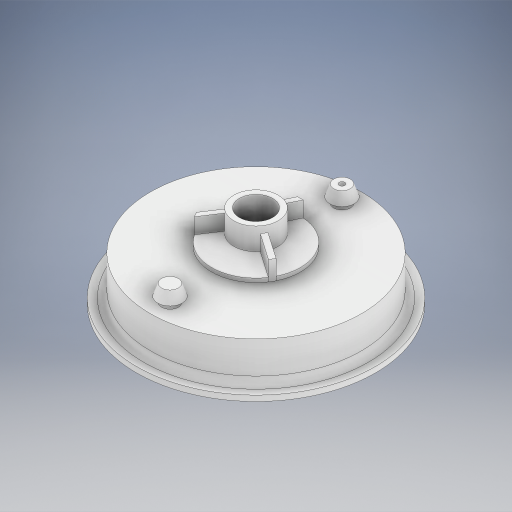
# Autodesk Inventor part: Pressure Plate
Saved by Autodesk Inventor 2024.1 (Build 281209000, 209)
## iProperties
Created: 2023-11-09
Part Number: Pressure Plate
Material: Acetal Resin, White
Document SubType Name: Modeling
Designer: Glen Collingwood
Density: 1.425 g/cm^3
Appearance: Smooth - White
Author: Glen Collingwood
Autodesk Inventor part; units mm, degrees
ref_plane "YZ Plane" through (0, 0, 0) normal (1, 0, 0) x (0, 1, 0)
ref_plane "XZ Plane" through (0, 0, 0) normal (0, 1, 0) x (-1, 0, 0)
ref_plane "XY Plane" through (0, 0, 0) normal (0, 0, 1) x (1, 0, 0)
sketch "Sketch1" plane through (0, 0, 0) normal (1, 0, 0) x (0, 1, 0)
  line L0 (0, 0) -> (0.5, 0)
  line L1 (0.5, 0) -> (0.5, -9.5)
  line L2 (0.5, -9.5) -> (0, -9.5)
  line L3 (0, -9.5) -> (0, 0)
  line L4 (0, 0) -> (-3.6315, 0)
  line L5 (0, -9.5) -> (-2.4, -9.5)
  line L6 (-3.5, -9.5) -> (-3.5, -9)
  line L7 (-2.4, -9) -> (0, -9)
  line L8 (0, -9) -> (0, -9.5)
  line L9 (-3.5, -9) -> (-3, -9)
  line L10 (-3, -10.1) -> (-3, -10.75)
  line L11 (-3, -10.75) -> (-3.5, -10.75)
  line L12 (-3.5, -10.75) -> (-3.5, -10.1)
  arc A0 (-2.4, -9.5) -> (-3, -10.1) centre (-2.4, -10.1) ccw
  arc A1 (-2.4, -9) -> (-3.5, -10.1) centre (-2.4, -10.1) ccw
  line L13 (0.5, -1.5) -> (-0.0667, -1.5)
  point P0 (-1.8158, 0)
  point P1 (0, -1.5)
  dimension "d0" = 19
  dimension "d1" = 0.5
  dimension "d2" = 4
  dimension "d3" = 0.5
  dimension "d4" = 0.5
  dimension "d5" = 21.5
  dimension "d6" = 0.6
  dimension "d7" = 1.1
  dimension "d8" = 3
  constraints: 28 end point, 6 parallel, 5 point on line, 4 horizontal, 4 perpendicular, 4 point on circle, 4 tangent, 2 centre point, 1 midpoint
  measures "d0" diameter of L2 point (-1.816, 0)
  measures "d1" distance of L1.end L2.end
  measures "d2" distance between parallel lines of L6 L1
  measures "d3" distance of L6.start L6.end
  measures "d4" distance of L10.end L11.end
  measures "d5" diameter of L11 L4
  measures "d6" radius of A0
  measures "d7" radius of A1
  measures "d8" diameter of L13 L4
revolve "Revolution1" add sketch "Sketch1" angle 360 about axis through (0, 0, 0) along (0, -1, 0) contours L13 L1 L2 L3 | L3 L5 A0 L10 L11 L12 A1 L7
sketch "Sketch2" plane through (0, 0, 0) normal (0, -1, 0) x (1, 0, 0)
  circle A0 centre (0, 0) radius 1.5 projected
  circle A1 centre (0, 0) radius 4.25
  circle A2 centre (0, 0) radius 4.5
  dimension "d10" = 8.5
  dimension "d11" = 9
  constraints: 2 centre point, 2 coincident
  measures "d10" diameter of A1
  measures "d11" diameter of A2
extrude "Extrusion1" add sketch "Sketch2" along normal blind 0.25 contours A2
sketch "Sketch3" plane through (0, 0.5, 0) normal (0, 1, 0) x (1, 0, 0)
  line L0 (0, 7.75) -> (0, -7.75)
  circle A0 centre (0, 7.75) radius 0.75
  circle A1 centre (0, -7.75) radius 0.75
  point P0 (0, 0)
  point P1 (0, 0)
  dimension "d14" = 15.5
  dimension "d15" = 1.5
  dimension "d16" = 1.5
  constraints: 3 coincident, 2 centre point, 2 end point, 1 midpoint, 1 vertical
  measures "d14" distance of L0.start L0.end
  measures "d15" diameter of A0
  measures "d16" diameter of A1
extrude "Extrusion2" add sketch "Sketch3" along normal blind 1.5
sketch "Sketch4" plane through (0, 0, 0) normal (1, 0, 0) x (0, 1, 0)
  line L0 (2, 7) -> (2, 8.5) projected
  line L1 (2, 7) -> (1, 6.65)
  line L2 (1, 6.65) -> (1, 7)
  line L3 (0.5, 9.5) -> (0.5, -9.5) projected
  line L4 (0.5, -9.5) -> (-2.4, -9.5) projected
  arc A0 (-2.4, -9.5) -> (-3, -10.1) centre (-2.4, -10.1) ccw projected
  line L5 (-3, -10.1) -> (-3, -10.75) projected
  line L6 (-3, -10.75) -> (-3.5, -10.75) projected
  line L7 (-3.5, -10.75) -> (-3.5, -10.1) projected
  arc A1 (-2.4, -9) -> (-3.5, -10.1) centre (-2.4, -10.1) ccw projected
  line L8 (-2.4, -9) -> (0, -9) projected
  line L9 (0, -9) -> (0, -4.5) projected
  line L10 (0, -4.5) -> (-0.25, -4.5) projected
  line L11 (-0.25, -4.5) -> (-0.25, -4.25) projected
  line L12 (-0.25, -4.25) -> (0, -4.25) projected
  line L13 (0, -4.25) -> (0, -1.5) projected
  line L14 (0, -1.5) -> (0.5, -1.5) projected
  line L15 (0.5, -1.5) -> (0.5, -7) projected
  line L16 (0.5, -7) -> (2, -7) projected
  line L17 (2, -7) -> (2, -8.5) projected
  line L18 (2, -8.5) -> (0.5, -8.5) projected
  line L19 (0.5, -8.5) -> (0.5, -9.5) projected
  line L20 (-2.4, 9.5) -> (0.5, 9.5) projected
  line L21 (0.5, 9.5) -> (0.5, 8.5) projected
  line L22 (0.5, 8.5) -> (2, 8.5) projected
  line L23 (2, 7) -> (0.5, 7) projected
  line L24 (0.5, 7) -> (0.5, 1.5) projected
  line L25 (0.5, 1.5) -> (0, 1.5) projected
  line L26 (0, 1.5) -> (0, 4.25) projected
  line L27 (0, 4.25) -> (-0.25, 4.25) projected
  line L28 (-0.25, 4.25) -> (-0.25, 4.5) projected
  line L29 (-0.25, 4.5) -> (0, 4.5) projected
  line L30 (0, 4.5) -> (0, 9) projected
  line L31 (0, 9) -> (-2.4, 9) projected
  arc A2 (-3.5, 10.1) -> (-2.4, 9) centre (-2.4, 10.1) ccw projected
  line L32 (-3.5, 10.1) -> (-3.5, 10.75) projected
  line L33 (-3.5, 10.75) -> (-3, 10.75) projected
  line L34 (-3, 10.75) -> (-3, 10.1) projected
  arc A3 (-3, 10.1) -> (-2.4, 9.5) centre (-2.4, 10.1) ccw projected
  line L35 (2, 7.75) -> (3.0151, 7.75)
  line L36 (2, 8.5) -> (2, 7) projected
  point P0 (0, 0)
  dimension "d19" = 0.5
  dimension "d20" = 0.35
  constraints: 6 end point, 1 horizontal, 1 midpoint, 1 parallel, 1 point on line
  measures "d19" distance between parallel lines of L3 L2
  measures "d20" distance of L1.end L2.end
revolve "Revolution2" add sketch "Sketch4" angle 360 about axis through (0, 2, 7.75) along (0, 1, 0) contours L1 L2 L23
mirror "Mirror1" about plane through (0, 0, 0) normal (0, 0, 1) of "Revolution2"
sketch "Sketch5" plane through (0, 2, -7.75) normal (0, 1, 0) x (1, 0, 0)
  circle A0 centre (0, 0) radius 0.75 projected
  circle A1 centre (0, -15.5) radius 0.75 projected
  point P0 (0, -7.75)
hole "Hole1" at (0, 2, -7.75) direction (0, -1, 0) diameter 0.5 end through all
sketch "Sketch6" plane through (0, 0, 0) normal (0, -1, 0) x (1, 0, 0)
  circle A0 centre (0, -7.75) radius 0.25 projected
  circle A1 centre (0, 0) radius 4.25 projected
  circle A2 centre (0, 0) radius 4.5 projected
  circle A3 centre (0, 0) radius 9 projected
  circle A4 centre (0, 0) radius 9.5 projected
  circle A5 centre (0, 0) radius 1.5 projected
  circle A6 centre (0, -7.75) radius 1.5
  point P0 (-0.8924, -8.9556)
  point P1 (0.8924, -8.9556)
  dimension "d29" = 3
  constraints: 1 centre point, 1 coincident
  measures "d29" diameter of A6
extrude "Extrusion3" add sketch "Sketch6" along normal blind 1.5 contours A6 A3 picked at (-0.4441, -8.6355)
chamfer "Chamfer1" distance 0.5 distance2 1 1 edges at (-0.25, -1.5, -7.75)
sketch "Sketch7" plane through (0, 0, 0) normal (1, 0, 0) x (0, 1, 0)
  line L0 (0, -4.5) -> (-0.25, -4.5) projected
  line L1 (-0.25, -4.5) -> (-0.25, -4.25) projected
  line L2 (-0.25, -4.25) -> (0, -4.25) projected
  line L3 (0, -4.25) -> (0, -1.5) projected
  line L4 (0, -1.5) -> (0.5, -1.5) projected
  line L5 (0.5, -1.5) -> (0.5, -7) projected
  line L6 (0.5, -7) -> (1, -7) projected
  line L7 (1, -7) -> (1, -6.65) projected
  line L8 (1, -6.65) -> (2, -7) projected
  line L9 (2, -7) -> (2, -7.5) projected
  line L10 (2, -7.5) -> (-0.5, -7.5) projected
  line L11 (-0.5, -7.5) -> (-1.5, -7) projected
  line L12 (-1.5, -7) -> (-1.5, -6.25) projected
  line L13 (-1.5, -6.25) -> (0, -6.25) projected
  line L14 (0, -6.25) -> (0, -4.5) projected
  line L15 (0.5, -9.5) -> (-2.4, -9.5) projected
  arc A0 (-2.4, -9.5) -> (-3, -10.1) centre (-2.4, -10.1) ccw projected
  line L16 (-3, -10.1) -> (-3, -10.75) projected
  line L17 (-3, -10.75) -> (-3.5, -10.75) projected
  line L18 (-3.5, -10.75) -> (-3.5, -10.1) projected
  arc A1 (-2.4, -9) -> (-3.5, -10.1) centre (-2.4, -10.1) ccw projected
  line L19 (-2.4, -9) -> (-1.5, -9) projected
  line L20 (-1.5, -9) -> (-1.5, -8.5) projected
  line L21 (-1.5, -8.5) -> (-0.5, -8) projected
  line L22 (-0.5, -8) -> (2, -8) projected
  line L23 (2, -8) -> (2, -8.5) projected
  line L24 (2, -8.5) -> (1, -8.85) projected
  line L25 (1, -8.85) -> (1, -8.5) projected
  line L26 (1, -8.5) -> (0.5, -8.5) projected
  line L27 (0.5, -8.5) -> (0.5, -9.5) projected
  line L28 (-2.4, 9.5) -> (0.5, 9.5) projected
  line L29 (0.5, 9.5) -> (0.5, 8.5) projected
  line L30 (0.5, 8.5) -> (1, 8.5) projected
  line L31 (1, 8.5) -> (1, 8.85) projected
  line L32 (1, 8.85) -> (2, 8.5) projected
  line L33 (2, 8.5) -> (2, 7) projected
  line L34 (2, 7) -> (1, 6.65) projected
  line L35 (1, 6.65) -> (1, 7) projected
  line L36 (1, 7) -> (0.5, 7) projected
  line L37 (0.5, 7) -> (0.5, 1.5) projected
  line L38 (0.5, 1.5) -> (0, 1.5) projected
  line L39 (0, 1.5) -> (0, 4.25) projected
  line L40 (0, 4.25) -> (-0.25, 4.25) projected
  line L41 (-0.25, 4.25) -> (-0.25, 4.5) projected
  line L42 (-0.25, 4.5) -> (0, 4.5) projected
  line L43 (0, 4.5) -> (0, 9) projected
  line L44 (0, 9) -> (-2.4, 9) projected
  arc A2 (-3.5, 10.1) -> (-2.4, 9) centre (-2.4, 10.1) ccw projected
  line L45 (-3.5, 10.1) -> (-3.5, 10.75) projected
  line L46 (-3.5, 10.75) -> (-3, 10.75) projected
  line L47 (-3, 10.75) -> (-3, 10.1) projected
  arc A3 (-3, 10.1) -> (-2.4, 9.5) centre (-2.4, 10.1) ccw projected
  line L48 (0.5, 1.5) -> (0.5, -1.5) projected
  line L49 (0.5, 0) -> (4, 0)
  line L50 (4, 0) -> (4, -4)
  line L51 (4, -4) -> (0.5, -4)
  line L52 (0.5, -4) -> (0.5, 0)
  line L53 (0.5, 0) -> (-1.5, 0)
  line L54 (-1.5, 0) -> (-1.5, -1.5)
  line L55 (-1.5, -1.5) -> (0.5, -1.5)
  line L56 (0.5, -1.5) -> (0.5, 0)
  line L57 (4, -2) -> (2, -2)
  line L58 (2, -2) -> (1.35, -4)
  line L59 (0.5, -1.5) -> (1, -1.5)
  line L60 (1, -1.5) -> (1, -4)
  line L61 (1, -4) -> (0.5, -4)
  line L62 (0.5, -4) -> (0.5, -1.5)
  line L63 (0, -1.75) -> (-1.5, -0.8)
  point P0 (0, 0)
  dimension "d35" = 4
  dimension "d36" = 3.5
  dimension "d37" = 2
  dimension "d38" = 0.85
  dimension "d39" = 2
  dimension "d40" = 0.5
  dimension "d41" = 1.5
  dimension "d42" = 0.8
  dimension "d43" = 0.25
  constraints: 30 end point, 6 parallel, 4 horizontal, 4 point on line, 3 perpendicular, 2 midpoint, 1 collinear
  measures "d35" distance from line of L51 point (0, 0)
  measures "d36" distance of L50.end L51.end
  measures "d37" distance between parallel lines of L57 L49
  measures "d38" distance from line of L58.end L5
  measures "d39" distance of L57.start L57.end
  measures "d40" distance between parallel lines of L5 L60
  measures "d41" distance between parallel lines of L54 L3
  measures "d42" distance from line of L63.end L53
  measures "d43" distance from line of L63.start L55
revolve "Revolution3" add sketch "Sketch7" angle 360 about axis through (0, 0.5, 0) along (0, 1, 0) separate body contours L63 L55 L3 | L55 L63 L54 L53 L48 L4 | L48 L49 L50 L57 L58 L51 L60 L59
sketch "Sketch8" plane through (0, 4, 0) normal (0, 1, 0) x (1, 0, 0)
  circle A0 centre (0, 0) radius 2 projected
  point P0 (0, 0)
hole "Hole2" at (0, 4, 0) direction (0, -1, 0) diameter 3 depth 3 tip angle 118 bodies 2
sketch "Sketch9" plane through (0, 0, 0) normal (1, 0, 0) x (0, 1, 0)
  line L0 (0, -4.5) -> (-0.25, -4.5) projected
  line L1 (-0.25, -4.5) -> (-0.25, -4.25) projected
  line L2 (-0.25, -4.25) -> (0, -4.25) projected
  line L3 (0, -4.25) -> (0, -1.5) projected
  line L4 (0, -1.5) -> (0.5, -1.5) projected
  line L5 (0.5, -1.5) -> (0.5, -7) projected
  line L6 (0.5, -7) -> (1, -7) projected
  line L7 (1, -7) -> (1, -6.65) projected
  line L8 (1, -6.65) -> (2, -7) projected
  line L9 (2, -7) -> (2, -7.5) projected
  line L10 (2, -7.5) -> (-0.5, -7.5) projected
  line L11 (-0.5, -7.5) -> (-1.5, -7) projected
  line L12 (-1.5, -7) -> (-1.5, -6.25) projected
  line L13 (-1.5, -6.25) -> (0, -6.25) projected
  line L14 (0, -6.25) -> (0, -4.5) projected
  line L15 (0.5, -9.5) -> (-2.4, -9.5) projected
  arc A0 (-2.4, -9.5) -> (-3, -10.1) centre (-2.4, -10.1) ccw projected
  line L16 (-3, -10.1) -> (-3, -10.75) projected
  line L17 (-3, -10.75) -> (-3.5, -10.75) projected
  line L18 (-3.5, -10.75) -> (-3.5, -10.1) projected
  arc A1 (-2.4, -9) -> (-3.5, -10.1) centre (-2.4, -10.1) ccw projected
  line L19 (-2.4, -9) -> (-1.5, -9) projected
  line L20 (-1.5, -9) -> (-1.5, -8.5) projected
  line L21 (-1.5, -8.5) -> (-0.5, -8) projected
  line L22 (-0.5, -8) -> (2, -8) projected
  line L23 (2, -8) -> (2, -8.5) projected
  line L24 (2, -8.5) -> (1, -8.85) projected
  line L25 (1, -8.85) -> (1, -8.5) projected
  line L26 (1, -8.5) -> (0.5, -8.5) projected
  line L27 (0.5, -8.5) -> (0.5, -9.5) projected
  line L28 (-2.4, 9.5) -> (0.5, 9.5) projected
  line L29 (0.5, 9.5) -> (0.5, 8.5) projected
  line L30 (0.5, 8.5) -> (1, 8.5) projected
  line L31 (1, 8.5) -> (1, 8.85) projected
  line L32 (1, 8.85) -> (2, 8.5) projected
  line L33 (2, 8.5) -> (2, 7) projected
  line L34 (2, 7) -> (1, 6.65) projected
  line L35 (1, 6.65) -> (1, 7) projected
  line L36 (1, 7) -> (0.5, 7) projected
  line L37 (0.5, 7) -> (0.5, 1.5) projected
  line L38 (0.5, 1.5) -> (0, 1.5) projected
  line L39 (0, 1.5) -> (0, 4.25) projected
  line L40 (0, 4.25) -> (-0.25, 4.25) projected
  line L41 (-0.25, 4.25) -> (-0.25, 4.5) projected
  line L42 (-0.25, 4.5) -> (0, 4.5) projected
  line L43 (0, 4.5) -> (0, 9) projected
  line L44 (0, 9) -> (-2.4, 9) projected
  arc A2 (-3.5, 10.1) -> (-2.4, 9) centre (-2.4, 10.1) ccw projected
  line L45 (-3.5, 10.1) -> (-3.5, 10.75) projected
  line L46 (-3.5, 10.75) -> (-3, 10.75) projected
  line L47 (-3, 10.75) -> (-3, 10.1) projected
  arc A3 (-3, 10.1) -> (-2.4, 9.5) centre (-2.4, 10.1) ccw projected
  line L48 (-1.5, -0.8) -> (-1.5, 0.8) projected
  line L49 (-1.5, 0.8) -> (0, 1.75) projected
  line L50 (0, 1.75) -> (0, 1.5) projected
  line L51 (0, 1.5) -> (1, 1.5) projected
  line L52 (1, 1.5) -> (1, 4) projected
  line L53 (1, 4) -> (1.35, 4) projected
  line L54 (1.35, 4) -> (2, 2) projected
  line L55 (2, 2) -> (4, 2) projected
  line L56 (4, 2) -> (4, 1.5) projected
  line L57 (4, 1.5) -> (1, 1.5) projected
  line L58 (1, 1.5) -> (0.0987, 0) projected
  line L59 (0.0987, 0) -> (1, -1.5) projected
  line L60 (1, -1.5) -> (4, -1.5) projected
  line L61 (4, -1.5) -> (4, -2) projected
  line L62 (4, -2) -> (2, -2) projected
  line L63 (2, -2) -> (1.35, -4) projected
  line L64 (1.35, -4) -> (1, -4) projected
  line L65 (1, -4) -> (1, -1.5) projected
  line L66 (1, -1.5) -> (0, -1.5) projected
  line L67 (0, -1.5) -> (0, -1.75) projected
  line L68 (0, -1.75) -> (-1.5, -0.8) projected
  line L69 (3.4, -2) -> (2.75, -4)
  line L70 (2.75, -4) -> (1, -4)
  line L71 (2, -2) -> (2, 2) projected
  line L72 (2, -2) -> (1, -2)
  point P0 (0, 0)
  dimension "d52" = 0.6
  constraints: 6 end point, 2 point on line, 1 horizontal, 1 parallel, 1 perpendicular
  measures "d52" distance from line of L69.start L61
extrude "Extrusion4" add sketch "Sketch9" along normal mid plane 0.5 contours L72 L63 L64 L65 | L62 L69 L70 L63 bodies 2
pattern_circular "Circular Pattern1" count 3 over 360 about axis through (0, 3, 0) along (0, 1, 0) of "Extrusion4" bodies 2
sketch "Sketch10" plane through (0, -1.5, 0) normal (0, -1, 0) x (1, 0, 0)
  circle A0 centre (0, -7.75) radius 0.75 projected
  arc A1 (-0.8924, -8.9556) -> (0.8924, -8.9556) centre (0, 0) ccw projected
  arc A2 (0.8924, -8.9556) -> (-0.8924, -8.9556) centre (0, -7.75) ccw projected
  arc A3 (0.8924, -8.9556) -> (-0.8924, -8.9556) centre (0, 0) ccw projected
  circle A4 centre (0, 0) radius 9.5 projected
  circle A5 centre (0, 0) radius 0.8 projected
  point P0 (0, 0)
hole "Hole3" at (0, -1.5, 0) direction (0, 1, 0) diameter 0.5 depth 30 bodies 2
equation "\"d3\" = d1"
equation "\"d4\" = d1"
body "Solid1"
body "Solid2"
